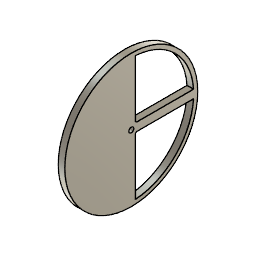
LED Box Hat (Autodesk Fusion 360 design; units mm, degrees)
Autodesk Fusion 360 part; units mm, degrees
sketch "Sketch1" plane through (0, 0, 0) normal (1, 0, 0) x (0, 1, 0)
  circle A0 centre (0, 0) radius 80
  dimension "d1" = 160
  constraint coincident A0.centre origin
  measures "d1" diameter of A0
extrude "Extrude1" add sketch "Sketch1" along normal blind 3 makes body 1
copy_body "Body->Comp1" bodies 1 removing the originals makes body 2 in component "Component"
sketch "Sketch2" plane through (3, 0, 0) normal (1, 0, 0) x (0, 1, 0)
  circle A0 centre (0, 0) radius 80
  circle A1 centre (0, 0) radius 3
  dimension "d4" = 6
  constraint concentric A0 A1
  measures "d4" diameter of A1
extrude "Extrude1'" cut sketch "Sketch2" against normal blind 10 contours A1 bodies 2 in component "Component"
sketch "Sketch3" plane through (3, 0, 0) normal (1, 0, 0) x (0, 1, 0)
  circle A0 centre (0, 0) radius 3
  circle A1 centre (0, 0) radius 80
  circle A2 centre (0, 0) radius 75
  circle A3 centre (0, 0) radius 8
  line L0 (-5, 77.486) -> (5, 77.486)
  line L1 (5, 77.486) -> (5, -77.486)
  line L2 (5, -77.486) -> (-5, -77.486)
  line L3 (-5, -77.486) -> (-5, 77.486)
  line L4 (-5, 77.486) -> (5, -77.486) construction
  line L5 (5, 77.486) -> (-5, -77.486) construction
  line L6 (-77.0993, 5) -> (77.0993, 5)
  line L7 (77.0993, 5) -> (77.0993, -5)
  line L8 (77.0993, -5) -> (-77.0993, -5)
  line L9 (-77.0993, -5) -> (-77.0993, 5)
  line L10 (-77.0993, 5) -> (77.0993, -5) construction
  line L11 (77.0993, 5) -> (-77.0993, -5) construction
  dimension "d7" = 150
  dimension "d8" = 16
  dimension "d9" = 10
  dimension "d10" = 10
  constraint coincident A0.centre A1.centre
  constraint concentric A2 A3
  constraint horizontal L0
  constraint perpendicular L0 L1
  constraint parallel L0 L2
  constraint parallel L1 L3
  constraint coincident L4 A0.centre
  constraint coincident L5 A0.centre
  constraint horizontal L6
  constraint perpendicular L6 L7
  constraint parallel L6 L8
  constraint parallel L7 L9
  constraint coincident L10 A0.centre
  constraint coincident L11 A0.centre
  measures "d7" diameter of A2
  measures "d8" diameter of A3
  measures "d9" distance of L1.end L2.end
  measures "d10" distance of L6.end L7.end
extrude "Extrude2" cut sketch "Sketch3" against normal blind 40 contours A2 A3 L1 L6 | A2 A3 L1 L8 bodies 2 in component "Component"
extrude "Extrude3" add 1 faces at (3, -2.6006, 53.0241) along direction (1, 0, 0) blind 5 on bodies 2 bodies 2 in component "Component"
component "Component" placed x (1, 0, 0) y (0, 1, 0) z (0, 0, 1) at (0, 0, 0)
